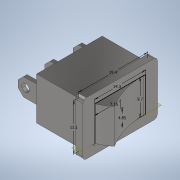
# Autodesk Inventor part: Rocker Switch
Saved by Autodesk Inventor 2023 (Build 270158000, 158)
## iProperties
Created: 2019-06-19
Part Number: Rocker Switch
Material: ABS Plastic
Document SubType Name: Modeling
Designer: pepd9
Density: 1.06 g/cm^3
Appearance: Steel - Polished
Author: pepd9
Autodesk Inventor part; units mm, degrees
ref_plane "YZ Plane" through (0, 0, 0) normal (1, 0, 0) x (0, 1, 0)
ref_plane "XZ Plane" through (0, 0, 0) normal (0, 1, 0) x (-1, 0, 0)
ref_plane "XY Plane" through (0, 0, 0) normal (0, 0, 1) x (1, 0, 0)
sketch "Sketch1" plane through (0, 0, 0) normal (1, 0, 0) x (0, 1, 0)
  line L0 (-7.5, 10.5) -> (7.5, 10.5)
  line L1 (7.5, 10.5) -> (7.5, -10.5)
  line L2 (7.5, -10.5) -> (-7.5, -10.5)
  line L3 (-7.5, -10.5) -> (-7.5, 10.5)
  point P0 (0, 0)
  dimension "d0" = 21
  dimension "d1" = 15
  dimension "d2" = 7.5
  dimension "d3" = 10.5
  constraints: 8 end point, 2 parallel, 1 horizontal, 1 perpendicular
  measures "d0" distance of L0.end L1.end
  measures "d1" distance of L1.end L2.end
  measures "d2" distance from line of L1 point (0, 0)
  measures "d3" distance from line of point (0, 0) L2
extrude "Extrusion1" add sketch "Sketch1" along normal blind 2
fillet "Fillet1" radius 1 4 edges at (1, -7.5, -10.5) (1, 7.5, -10.5) (1, 7.5, 10.5) (1, -7.5, 10.5)
sketch "Sketch2" plane through (2, 0, 0) normal (1, 0, 0) x (0, 0, -1)
  line L0 (-7.15, 4.85) -> (7.15, 4.85)
  line L1 (7.15, 4.85) -> (7.15, -4.85)
  line L2 (7.15, -4.85) -> (-7.15, -4.85)
  line L3 (-7.15, -4.85) -> (-7.15, 4.85)
  point P0 (0, 0)
  dimension "d7" = 4.85
  dimension "d8" = 9.7
  dimension "d9" = 14.3
  dimension "d10" = 7.15
  constraints: 8 end point, 2 parallel, 1 coincident, 1 horizontal, 1 perpendicular
  measures "d7" distance from line of point (0, 0) L2
  measures "d8" distance of L0.end L1.end
  measures "d9" distance of L0.start L0.end
  measures "d10" distance from line of point (0, 0) L3
ref_plane "Work Plane1" through (2, -4.85, 7.15) normal (0, -1, 0) x (1, 0, 0)
sketch "Sketch3" plane through (2, -4.85, 7.15) normal (0, -1, 0) x (1, 0, 0)
  arc A0 (3.5, -2.0473) -> (0, 0) centre (-3.3399, -9.7251) ccw
  line L0 (0, -16.65) -> (0, 2.35) projected
  arc A1 (3.5, -2.0473) -> (0, -14.3) centre (22.3145, -14.0479) ccw
  point P0 (-2, -7.15)
  point P1 (0, -13.7959)
  dimension "d11" = 3.5
  constraints: 4 point on circle, 2 centre point
  measures "d11" distance from line of L0 A0.start
extrude "Extrusion2" add sketch "Sketch3" against normal blind 9.7
sketch "Sketch4" plane through (0, 0, 0) normal (-1, 0, 0) x (0, 0, 1)
  line L0 (9.25, -6) -> (-9.25, -6)
  line L1 (-9.25, -6) -> (-9.25, 6)
  line L2 (-9.25, 6) -> (9.25, 6)
  line L3 (9.25, 6) -> (9.25, -6)
  line L4 (9.5, -7.5) -> (-9.5, -7.5) projected
  line L5 (10.5, 6.5) -> (10.5, -6.5) projected
  point P0 (0, 0)
  dimension "d14" = 18.5
  dimension "d15" = 12
  dimension "d16" = 1.5
  dimension "d17" = 1.25
  constraints: 8 end point, 2 parallel, 1 horizontal, 1 perpendicular
  measures "d14" distance of L1.end L2.end
  measures "d15" distance of L0.end L1.end
  measures "d16" distance between parallel lines of L4 L0
  measures "d17" distance between parallel lines of L5 L3
extrude "Extrusion3" add sketch "Sketch4" along normal blind 12.3
sketch "Sketch5" plane through (-12.3, 0, 0) normal (-1, 0, 0) x (0, 0, 1)
  line L0 (9.25, -6) -> (9.25, 6) projected
  line L1 (-9.25, -6) -> (-9.25, 6) projected
  line L2 (9.25, 2.5) -> (-9.25, 2.5)
  line L3 (-9.25, 2.5) -> (-9.25, -2.5)
  line L4 (-9.25, -2.5) -> (9.25, -2.5)
  line L5 (9.25, -2.5) -> (9.25, 2.5)
  line L6 (9.25, 6) -> (-9.25, 6) projected
  point P0 (0, 0)
  point P1 (9.25, -2.5)
  point P2 (-9.25, 2.5)
  dimension "d20" = 5
  dimension "d21" = 3.5
  constraints: 8 end point, 2 parallel, 2 point on line, 1 horizontal, 1 perpendicular
  measures "d20" distance between parallel lines of L2 L4
  measures "d21" distance between parallel lines of L6 L2
extrude "Extrusion4" add sketch "Sketch5" along normal blind 6.2 contours L4 L1 L2 L0
sketch "Sketch6" plane through (-18.5, 0, 0) normal (-1, 0, 0) x (0, 0, 1)
  line L0 (9.25, 2.5) -> (-9.25, 2.5) projected
  line L1 (-9.25, 2.5) -> (-9.25, -2.5) projected
  line L2 (-9.25, -2.5) -> (9.25, -2.5) projected
  line L3 (9.25, -2.5) -> (9.25, 2.5) projected
  line L4 (9.25, 2.5) -> (8.25, 2.5)
  line L5 (8.25, 2.5) -> (8.25, -2.5)
  line L6 (8.25, -2.5) -> (9.25, -2.5)
  line L7 (9.25, -2.5) -> (9.25, 2.5)
  line L8 (7.25, -2.5) -> (0.75, -2.5)
  line L9 (0.75, -2.5) -> (0.75, 2.5)
  line L10 (0.75, 2.5) -> (7.25, 2.5)
  line L11 (7.25, 2.5) -> (7.25, -2.5)
  line L12 (-9.25, 2.5) -> (9.25, 2.5) projected
  line L13 (-7.25, -2.5) -> (-0.25, -2.5)
  line L14 (-0.25, -2.5) -> (-0.25, 2.5)
  line L15 (-0.25, 2.5) -> (-7.25, 2.5)
  line L16 (-7.25, 2.5) -> (-7.25, -2.5)
  line L17 (9.25, -2.5) -> (-9.25, -2.5) projected
  line L18 (-9.25, 2.5) -> (-8.25, 2.5)
  line L19 (-8.25, 2.5) -> (-8.25, -2.5)
  line L20 (-8.25, -2.5) -> (-9.25, -2.5)
  line L21 (-9.25, -2.5) -> (-9.25, 2.5)
  point P0 (0, 0)
  point P1 (-8.25, -2.5)
  point P2 (-0.25, -2.5)
  point P3 (7.25, 2.5)
  dimension "d24" = 1
  dimension "d25" = 1
  dimension "d26" = 1
  dimension "d27" = 1
  dimension "d28" = 1
  dimension "d29" = 6.5
  constraints: 32 end point, 8 parallel, 5 point on line, 4 horizontal, 4 perpendicular, 2 other
  measures "d24" distance between parallel lines of L1 L19
  measures "d25" distance between parallel lines of L16 L19
  measures "d26" distance between parallel lines of L9 L14
  measures "d27" distance between parallel lines of L5 L11
  measures "d28" distance between parallel lines of L7 L5
  measures "d29" distance between parallel lines of L9 L11
extrude "Extrusion5" cut sketch "Sketch6" against normal blind 6.2 contours L3 L2 L5 L0 | L11 L2 L9 L0 | L14 L2 L16 L0 | L19 L2 L1 L0
chamfer "Chamfer1" distance 1.5 angle 45 6 edges at (-18.5, 2.5, -7.75) (-18.5, -2.5, -7.75) (-18.5, -2.5, 0.25) (-18.5, 2.5, 0.25) (-18.5, -2.5, 7.75) (-18.5, 2.5, 7.75)
sketch "Sketch7" plane through (-12.3, -2.5, -8.25) normal (0, 0, -1) x (-1, 0, 0)
  line L0 (6.2, 1.5) -> (4.7, 0) projected
  line L1 (6.2, 3.5) -> (6.2, 1.5) projected
  line L2 (4.7, 5) -> (6.2, 3.5) projected
  line L3 (0, 5) -> (4.7, 5) projected
  line L4 (0, 5) -> (0, 0) projected
  line L5 (4.7, 0) -> (0, 0) projected
  point P0 (-12.3, 2.5)
  point P1 (5.2, 2.5)
  point P2 (4.1377, 2.5)
hole "Hole1" at (-16.4377, 0, -8.25) direction (0, 0, 1) diameter 2.2 end through all
sketch "Sketch8" plane through (0, 0, 0) normal (-1, 0, 0) x (0, 0, 1)
  line L0 (-9.7, -6.55) -> (9.7, -6.55)
  line L1 (9.7, -6.55) -> (9.7, 6.55)
  line L2 (9.7, 6.55) -> (-9.7, 6.55)
  line L3 (-9.7, 6.55) -> (-9.7, -6.55)
  line L4 (-9.7, -6.55) -> (9.7, 6.55) construction
  line L5 (9.7, -6.55) -> (-9.7, 6.55) construction
  point P0 (0, 0)
  dimension "d42" = 19.4
  dimension "d43" = 13.1
  constraints: 12 end point, 2 midpoint, 2 parallel, 1 horizontal, 1 perpendicular
  measures "d42" distance of L2.end L1.end
  measures "d43" distance of L1.end L0.end
body "Solid1"
